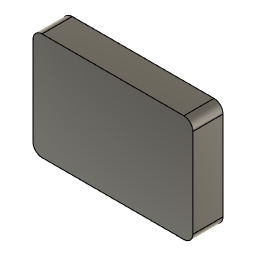
dice v1 (Autodesk Fusion 360 design; units mm, degrees)
Autodesk Fusion 360 part; units mm, degrees
sketch "Pico-Dice_2024-02-11" plane through (0, 0, 0) normal (0, 1, 0) x (1, 0, 0)
  line L0 (0, -5) -> (0, -54)
  line L1 (6, -60) -> (90, -60)
  line L2 (96, -54) -> (96, -5)
  line L3 (90, 1) -> (6, 1)
  circle A0 centre (3, -57) radius 1.5
  circle A1 centre (3, -2) radius 1.5
  circle A2 centre (93, -2) radius 1.5
  circle A3 centre (93, -56.952) radius 1.5
  line L4 (-0.5, 1.5) -> (-0.5, -60.5)
  line L5 (-0.5, -60.5) -> (96.5, -60.5)
  line L6 (96.5, -60.5) -> (96.5, 1.5)
  line L7 (96.5, 1.5) -> (-0.5, 1.5)
  line L8 (1, -65) -> (95, -65)
  line L9 (101, -59) -> (101, 0)
  line L10 (95, 6) -> (1, 6)
  line L11 (-5, 0) -> (-5, -59)
  arc A4 (-5, -59) -> (1, -65) centre (1, -59) ccw
  arc A5 (95, -65) -> (101, -59) centre (95, -59) ccw
  arc A6 (1, 6) -> (-5, 0) centre (1, 0) ccw
  arc A7 (101, 0) -> (95, 6) centre (95, 0) ccw
  line L12 (6, -60) -> (6, -54)
  line L13 (6, -54) -> (0, -54)
  line L14 (48, -65) -> (48, 6)
  line L15 (-5, -29.5) -> (101, -29.5)
  line L16 (90, -60) -> (90, -54)
  line L17 (90, -54) -> (96, -54)
  line L18 (6, 1) -> (6, -5)
  line L19 (6, -5) -> (0, -5)
  line L20 (90, -5) -> (96, -5)
  line L21 (90, 1) -> (90, -5)
  line L22 (6, 1) -> (6, 1.5)
  line L23 (-0.5, 1.5) -> (6, 1.5)
  line L24 (0, -5) -> (-0.5, -5)
  line L25 (-0.5, 1.5) -> (-0.5, -5)
  line L26 (90, 1) -> (90, 1.5)
  line L27 (96, -5) -> (96.5, -5)
  line L28 (96.5, 1.5) -> (90, 1.5)
  line L29 (90, -60) -> (90, -60.5)
  line L30 (96, -54) -> (96.5, -54)
  line L31 (96.5, -54) -> (96.5, -60.5)
  line L32 (6, -60) -> (6, -60.5)
  line L33 (6, -60.5) -> (-0.5, -60.5)
  line L34 (0, -54) -> (-0.5, -54)
  line L35 (-0.5, -54) -> (-0.5, -60.5)
  dimension "d3" = 6
  dimension "d4" = 6
  dimension "d5" = 6
  constraint tangent L8 A4
  constraint tangent L11 A4
  constraint tangent L8 A5
  constraint tangent L9 A5
  constraint equal A4 A5
  constraint tangent L11 A6
  constraint tangent L10 A6
  constraint equal A4 A6
  constraint tangent L9 A7
  constraint tangent L10 A7
  constraint equal A4 A7
  constraint vertical L12
  constraint horizontal L13
  constraint midpoint L8 L14.start
  constraint midpoint L10 L14.end
  constraint midpoint L11 L15.start
  constraint midpoint L9 L15.end
  constraint symmetric L1.start L14 L1.end
  constraint symmetric L12.end L14 L16.end
  constraint symmetric L0.end L14 L2.start
  constraint symmetric L1.start L15 L3.end
  constraint symmetric L12.end L15 L18.end
  constraint symmetric L0.end L15 L0.start
  constraint symmetric L15 L1.end L3.start
  constraint symmetric L15 L16.end L20.start
  constraint symmetric L15 L2.start L2.end
  constraint coincident L7 L22.end
  constraint perpendicular L7 L22
  constraint coincident L4 L24.end
  constraint perpendicular L4 L24
  constraint coincident L7 L26.end
  constraint perpendicular L7 L26
  constraint coincident L6 L27.end
  constraint perpendicular L6 L27
  measures "d3" radius of A4
  measures "d4" distance of L12.end L0.end
  measures "d5" distance of L1.start L12.end
extrude "Extrude1" add sketch "Pico-Dice_2024-02-11" along normal blind 20 contours L4 L7 L10 L11 A6 L14 L15 L23 L25 | L4 L5 L8 L11 A4 L14 L15 L33 L35 | L5 L6 L8 L9 A5 L14 L15 L31 | L6 L7 L9 L10 A7 L14 L15 L28
extrude "Extrude2" add sketch "Pico-Dice_2024-02-11" along normal blind 2 contours L0 L3 L14 L15 L18 L19 | L4 L7 L18 L19 L22 L23 L24 L25 | L0 L4 L15 L24 | L0 L1 L12 L13 L14 L15 | L0 L4 L15 L34 | L4 L5 L12 L13 L32 L33 L34 L35 | L1 L2 L14 L15 L16 L17 | L2 L3 L14 L15 L20 L21 | L3 L7 L14 L22 | L1 L5 L14 L32 | L1 L5 L14 L29 | L3 L7 L14 L26 | L2 L6 L15 L30 | L2 L6 L15 L27 | L5 L6 L16 L17 L29 L30 L31 | L6 L7 L20 L21 L26 L27 L28 | A0 | A1 | A2 | A3
extrude "Extrude3" add sketch "Pico-Dice_2024-02-11" along normal blind 10 contours L0 L3 L14 L15 L18 L19 | L0 L1 L12 L13 L14 L15 | L1 L2 L14 L15 L16 L17 | L2 L3 L14 L15 L20 L21 | A0 | A1 | A2 | A3
extrude "Extrude4" cut sketch "Pico-Dice_2024-02-11" along normal blind 30 from surface at 3 contours A0 | A1 | A2 | A3
extrude "Extrude5" add sketch "Pico-Dice_2024-02-11" along normal blind 10 contours L4 L7 L18 L19 L22 L23 L24 L25 | L4 L5 L12 L13 L32 L33 L34 L35 | L5 L6 L16 L17 L29 L30 L31 | L6 L7 L20 L21 L26 L27 L28
extrude "Extrude6" cut sketch "Pico-Dice_2024-02-11" along normal blind 21 from surface at 5 contours L0 L3 L14 L15 L18 L19 | L0 L1 L12 L13 L14 L15 | L1 L2 L14 L15 L16 L17 | L2 L3 L14 L15 L20 L21
extrude "Extrude7" cut 1 faces at (34, 5, 21.3333) along direction (0, -1, 0) blind 3
